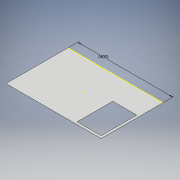
# Autodesk Inventor part: frontPanel
Saved by Autodesk Inventor 2017 (Build 210142000, 142)
## iProperties
Created: 2017-06-07
Part Number: frontPanel
Material: Generic
Document SubType Name: Sheet Metal
Designer: Roko
Density: 1 g/cm^3
Sheet Metal Rule: Default_mm
Appearance: Default
Author: Roko
Autodesk Inventor part; units mm, degrees
ref_plane "YZ Plane" through (0, 0, 0) normal (1, 0, 0) x (0, 1, 0)
ref_plane "XZ Plane" through (0, 0, 0) normal (0, 1, 0) x (-1, 0, 0)
ref_plane "XY Plane" through (0, 0, 0) normal (0, 0, 1) x (1, 0, 0)
sketch "Sketch1" plane through (0, 0, 0) normal (0, 0, 1) x (1, 0, 0)
  line L0 (-200, -130) -> (200, -130)
  line L1 (200, -130) -> (200, 130)
  line L2 (200, 130) -> (-200, 130)
  line L3 (-200, 130) -> (-200, -130)
  line L4 (-200, -130) -> (200, 130) construction
  line L5 (200, -130) -> (-200, 130) construction
  point P0 (0, 0)
  dimension "d0" = 400
  dimension "d1" = 260
  measures "d0" distance of L2.end L1.end
  measures "d1" distance of L1.end L0.end
extrude "Plate1" add sketch "Sketch1" along normal blind 0.5
sketch "Sketch2" plane through (0, 0, 0.5) normal (0, 0, 1) x (1, 0, 0)
  line L0 (-190, -120) -> (190, -120)
  line L1 (190, -120) -> (190, 120)
  line L2 (190, 120) -> (-190, 120)
  line L3 (-190, 120) -> (-190, -120)
  line L4 (-190, -120) -> (190, 120) construction
  line L5 (190, -120) -> (-190, 120) construction
  line L6 (-190, -120) -> (54, -120)
  line L7 (54, -120) -> (54, 124)
  line L8 (54, 124) -> (-190, 124)
  line L9 (-190, 124) -> (-190, -120)
  line L10 (190, -120) -> (89, -120)
  line L11 (89, -120) -> (89, 30)
  line L12 (89, 30) -> (190, 30)
  line L13 (190, 30) -> (190, -120)
  point P0 (0, 0)
  dimension "d3" = 380
  dimension "d4" = 240
  dimension "d5" = 244
  dimension "d6" = 244
  dimension "d7" = 101
  dimension "d8" = 150
  constraints: 28 end point, 6 parallel, 3 horizontal, 3 perpendicular, 2 midpoint
  measures "d3" distance of L2.end L1.end
  measures "d4" distance of L1.end L0.end
  measures "d5" distance of L8.end L7.end
  measures "d6" distance of L7.end L6.end
  measures "d7" distance of L11.end L12.end
  measures "d8" distance of L10.end L11.end
extrude "Cut1" cut sketch "Sketch2" against normal blind 0.5 contours L11 L12 L1 L0
sketch "Sketch3" plane through (0, 0, 0.5) normal (0, 0, 1) x (1, 0, 0)
  line L0 (-200, 130) -> (200, 130) projected
  point P0 (0, 0)
  dimension "d11" = 400
  measures "d11" distance of L0.start L0.end
sketch "Sketch4" plane through (0, 0, 0.5) normal (0, 0, 1) x (1, 0, 0)
  point P0 (0, 0)
equation "\"d9\" = Thickness"
equation "\"BendRadius\" = Thickness"
equation "\"BendReliefWidth\" = Thickness"
equation "\"BendReliefDepth\" = 0.5 * Thickness"
equation "\"CornerReliefSize\" = 4 * Thickness"
equation "\"MinimumRemnant\" = 2 * Thickness"
equation "\"TransitionRadius\" = BendRadius"
equation "\"JacobiRadiusSize\" = BendRadius"
equation "\"GapSize\" = Thickness"
equation "\"d2\" = BendRadius"
equation "\"Thickness\" = 0.5"
body "Solid1"
